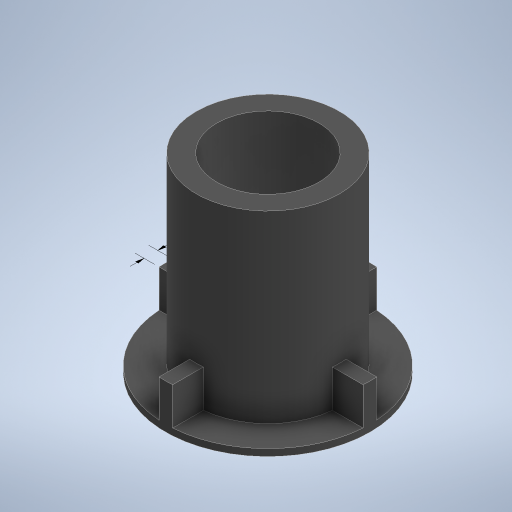
# Autodesk Inventor part: axis_in
Saved by Autodesk Inventor 2024.1 (Build 281209000, 209)
## iProperties
Created: 2024-04-01
Part Number: axis_in
Material: 一般
Document SubType Name: Modeling
Designer: hibik
Density: 1 g/cm^3
Appearance: 既定
Author: hibik
Autodesk Inventor part; units mm, degrees
ref_plane "YZ Plane" through (0, 0, 0) normal (1, 0, 0) x (0, 1, 0)
ref_plane "XZ Plane" through (0, 0, 0) normal (0, 1, 0) x (-1, 0, 0)
ref_plane "XY Plane" through (0, 0, 0) normal (0, 0, 1) x (1, 0, 0)
sketch "スケッチ1" plane through (0, 0, 0) normal (0, 1, 0) x (-1, 0, 0)
  circle A0 centre (0, 0) radius 15
  dimension "d0" = 30
  constraints: 1 centre point, 1 coincident
  measures "d0" diameter of A0
extrude "押し出し1" add sketch "スケッチ1" along normal blind 1
sketch "スケッチ2" plane through (0, 1, 0) normal (0, 1, 0) x (1, 0, 0)
  circle A0 centre (0, 0) radius 10.5
  dimension "d3" = 21
  constraints: 1 centre point, 1 coincident
  measures "d3" diameter of A0
extrude "押し出し2" add sketch "スケッチ2" along normal blind 27
ref_plane "作業平面1" through (0, 6, 0) normal (0, 1, 0) x (1, 0, 0)
sketch "スケッチ5" plane through (0, 1, 0) normal (0, 1, 0) x (1, 0, 0)
  line L0 (-15, 1) -> (-8.9813, 1)
  line L1 (-8.9813, 1) -> (-8.9813, -1)
  line L2 (-8.9813, -1) -> (-15, -1)
  line L3 (-15, -1) -> (-15, 1)
  circle A0 centre (0, 0) radius 15 projected
  circle A1 centre (0, 0) radius 15
  point P0 (-15, 0)
  point P1 (-14.9666, 1)
  point P2 (-14.9666, -1)
  point P3 (-14.9666, 1)
  point P4 (-14.9666, -1)
  dimension "d11" = 2
  dimension "d14" = 30
  constraints: 8 end point, 2 parallel, 1 centre point, 1 coincident, 1 horizontal, 1 horizontal alignment, 1 midpoint, 1 perpendicular, 1 tangent
  measures "d11" distance of L2.end L0.start
  measures "d14" diameter of A1
extrude "押し出し4" add sketch "スケッチ5" along normal blind 5.5 contours L0 L1 L2 A0 picked at (-10.9875, 0)
pattern_circular "円形状パターン1" count 4 over 360 about axis through (0, -10, 0) along (0, 1, 0) of "押し出し4"
sketch "スケッチ9" plane through (0, 0, 0) normal (0, -1, 0) x (1, 0, 0)
  circle A0 centre (0, 0) radius 7.5
  dimension "d40" = 15
  constraints: 1 centre point, 1 coincident
  measures "d40" diameter of A0
extrude "押し出し7" cut sketch "スケッチ9" against normal through all
